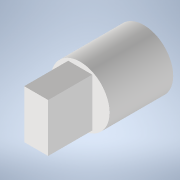
# Autodesk Inventor part: AdapterPoti2
Saved by Autodesk Inventor 2020.3 (Build 243373010, 373A)
## iProperties
Created: 2020-11-30
Part Number: AdapterPoti2
Material: Generisch
Document SubType Name: Modeling
Designer: Stefan
Density: 1 g/cm^3
Appearance: Vorgabe
Author: Stefan
Autodesk Inventor part; units mm, degrees
ref_plane "YZ Plane" through (0, 0, 0) normal (1, 0, 0) x (0, 1, 0)
ref_plane "XZ Plane" through (0, 0, 0) normal (0, 1, 0) x (-1, 0, 0)
ref_plane "XY Plane" through (0, 0, 0) normal (0, 0, 1) x (1, 0, 0)
sketch "Skizze1" plane through (0, 0, 0) normal (0, 0, 1) x (1, 0, 0)
  line L0 (-2.6557, -1.5) -> (2.6557, -1.5)
  circle A0 centre (0, 0) radius 6
  arc A1 (2.6557, -1.5) -> (-2.6557, -1.5) centre (0, 0) ccw
  dimension "d3" = 12
  dimension "d6" = 6.1
  constraints: 2 centre point, 2 end point, 2 point on circle, 1 coincident
  measures "d3" diameter of A0
  measures "d6" diameter of A1
extrude "Extrusion1" add sketch "Skizze1" along normal blind 11
sketch "Skizze4" plane through (0, 0, 11) normal (0, 0, 1) x (1, 0, 0)
  circle A0 centre (0, 0) radius 6
  dimension "d14" = 12
  constraints: 1 centre point, 1 coincident
  measures "d14" diameter of A0
extrude "Extrusion3" add sketch "Skizze4" along normal blind 2
sketch "Skizze5" plane through (0, 0, 13) normal (0, 0, 1) x (1, 0, 0)
  line L0 (-2.45, 4.95) -> (2.45, 4.95)
  line L1 (2.45, 4.95) -> (2.45, -4.95)
  line L2 (2.45, -4.95) -> (-2.45, -4.95)
  line L3 (-2.45, -4.95) -> (-2.45, 4.95)
  point P0 (0, 0)
  point P1 (0, 0)
  dimension "d17" = 4.9
  dimension "d18" = 9.9
  dimension "d19" = 2.45
  dimension "d20" = 4.95
  constraints: 8 end point, 2 parallel, 1 horizontal, 1 perpendicular
  measures "d17" distance of L1.end L2.end
  measures "d18" distance of L0.end L1.end
  measures "d19" distance from line of point (0, 0) L1
  measures "d20" distance from line of L0 point (0, 0)
extrude "Extrusion4" add sketch "Skizze5" along normal blind 9
